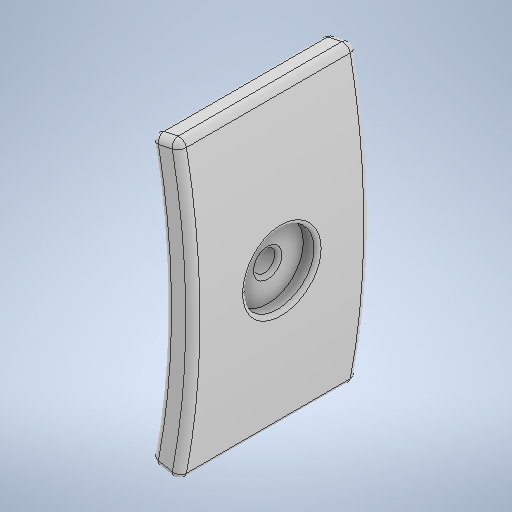
# Autodesk Inventor part: Pedal 2
Saved by Autodesk Inventor 2025.2 (Build 292293000, 293)
## iProperties
Created: 2025-03-16
Part Number: Pedal 2
Material: Generic
Document SubType Name: Modeling
Designer: eason
Density: 1 g/cm^3
Appearance: Default
Author: eason
Autodesk Inventor part; units mm, degrees
ref_plane "YZ Plane" through (0, 0, 0) normal (1, 0, 0) x (0, 1, 0)
ref_plane "XZ Plane" through (0, 0, 0) normal (0, 1, 0) x (-1, 0, 0)
sketch "Sketch1" plane through (0, 0, 0) normal (0, 0, 1) x (1, 0, 0)
  line L0 (0, 25) -> (0, -25)
  line L1 (-235.0313, 0) -> (56.1687, 0) projected
  line L2 (0, -58.24) -> (0, 58.24) projected
  line L3 (0, 25) -> (5, 25)
  line L4 (0, -25) -> (5, -25)
  arc A0 (2.5278, -40) -> (2.5278, 40) centre (-193.4313, 0) ccw
  line L5 (2.5278, 40) -> (10.3662, 41.6)
  line L6 (2.5278, -40) -> (10.3662, -41.6)
  arc A1 (10.3662, -41.6) -> (10.3662, 41.6) centre (-193.4313, 0) ccw
  point P0 (0, 0)
  point P1 (0, 0)
  point P2 (6.5687, 0)
  dimension "d0" = 50
  dimension "d1" = 5
  dimension "d2" = 200
  dimension "d3" = 80
  dimension "d4" = 8
  dimension "d27" = 23.074
  constraints: 10 end point, 7 point on circle, 4 line through centre, 2 centre point, 2 horizontal, 2 point on line, 1 collinear, 1 concentric, 1 midpoint, 1 parallel, 1 vertical
  measures "d0" distance of L0.start L0.end
  measures "d1" distance of L0.start L3.end
  measures "d2" radius of A0
  measures "d3" distance of L6.start L5.start
  measures "d4" radial gap between concentric circles of A1 A0
  measures "d27" angle of L6 L5
extrude "Extrusion1" add sketch "Sketch1" along normal mid plane 30 contours L3 A0 L1 L0 | L1 A0 L4 L0
extrude "Extrusion2" add sketch "Sketch1" along normal mid plane 50 contours A0 L5 A1 L1 | L1 A1 L6 A0
sketch "Sketch2" plane through (0, -25, 15) normal (-1, 0, 0) x (0, 0, 1)
  circle A0 centre (-15, 25) radius 3
  line L0 (-30, 0) -> (-30, 50) projected
  line L1 (-30, 25) -> (0, 25) construction
  line L2 (0, 50) -> (0, 0) projected
  line L3 (-30, 50) -> (0, 50) projected
  line L4 (-15, 50) -> (-15, 0) construction
  line L5 (-30, 0) -> (0, 0) projected
  dimension "d9" = 6
  constraints: 6 midpoint, 4 end point, 1 centre point
  measures "d9" diameter of A0
extrude "Extrusion3" cut sketch "Sketch2" against normal through all contours A0
sketch "Sketch3" plane through (0, -25, 15) normal (-1, 0, 0) x (0, 0, 1)
  line L0 (-27.2, 47.2) -> (-2.8, 47.2)
  line L1 (-2.8, 47.2) -> (-2.8, 2.8)
  line L2 (-2.8, 2.8) -> (-27.2, 2.8)
  line L3 (-27.2, 2.8) -> (-27.2, 47.2)
  line L4 (-30, 0) -> (-30, 50) projected
  line L5 (-30, 50) -> (0, 50) projected
  line L6 (0, 50) -> (0, 0) projected
  line L7 (-30, 0) -> (0, 0) projected
  line L8 (-23.8, 43.8) -> (-6.2, 43.8)
  line L9 (-6.2, 43.8) -> (-6.2, 6.2)
  line L10 (-6.2, 6.2) -> (-23.8, 6.2)
  line L11 (-23.8, 6.2) -> (-23.8, 43.8)
  point P0 (-15, 25)
  dimension "d13" = 2.8
  dimension "d14" = 2.8
  dimension "d15" = 2.8
  dimension "d16" = 2.8
  dimension "d17" = 3.4
  dimension "d18" = 3.4
  dimension "d19" = 3.4
  dimension "d20" = 3.4
  constraints: 16 end point, 4 parallel, 2 horizontal, 2 perpendicular
  measures "d13" distance between parallel lines of L4 L3
  measures "d14" distance between parallel lines of L5 L0
  measures "d15" distance between parallel lines of L6 L1
  measures "d16" distance between parallel lines of L7 L2
  measures "d17" distance between parallel lines of L8 L0
  measures "d18" distance between parallel lines of L2 L10
  measures "d19" distance between parallel lines of L1 L9
  measures "d20" distance between parallel lines of L3 L11
extrude "Extrusion4" cut sketch "Sketch3" against normal blind 3.2 contours L0 L1 L2 L3
ref_plane "Work Plane2" through (14.5687, 0, 0) normal (-1, 0, 0) x (0, 0, 1)
sketch "Sketch6" plane through (14.5687, 0, 0) normal (-1, 0, 0) x (0, 0, 1)
  circle A0 centre (0, 0) radius 10
  circle A1 centre (0, 0) radius 3 projected
  point P0 (0, 0)
  point P1 (0, 3)
  point P2 (0, -9.5)
  dimension "d34" = 20
  constraints: 1 centre point, 1 vertical alignment, 2 other
  measures "d34" diameter of A0
extrude "Extrusion6" cut sketch "Sketch6" along normal blind 4 contours A0 | A1
fillet "Fillet1" radius 2 4 edges at (6.447, -40.8, 25) (6.447, -40.8, -25) (6.447, 40.8, -25) (6.447, 40.8, 25)
fillet "Fillet2" radius 2 12 edges at (2.6249, 39.5214, -24.3096) (2.5278, 40, 0) (2.6249, 39.5214, 24.3096) (6.5687, 0, 25) (2.6249, -39.5213, 24.3096) (2.5278, -40, 0) (2.6249, -39.5213, -24.3096) (6.5687, 0, -25) (10.3662, -41.6, 0) (10.3662, 41.6, 0) (14.5687, 0, -25) (14.5687, 0, 25)
fillet "Fillet3" radius 1 4 edges at (10.5687, 0, -3) (0, 0, -3) (14.3281, 10, 0.0126) (14.3281, -10, 0.0124)
fillet "Fillet4" radius 1 12 edges at (0, 18.8, 0) (0, 0, 8.8) (0, 0, -8.8) (0, -18.8, 0) (0, 0, -15) (0, 0, -12.2) (0, -25, 0) (0, -22.2, 0) (0, 0, 12.2) (0, 0, 15) (0, 22.2, 0) (0, 25, 0)
body "Solid1"
